wireHolder v1 (Autodesk Fusion 360 design; units mm, degrees)
Autodesk Fusion 360 part; units mm, degrees
sketch "Sketch1" plane through (0, 0, 0) normal (0, 0, 1) x (1, 0, 0)
  line L0 (0, 0) -> (40, 0)
  line L1 (40, 0) -> (40, 20)
  line L2 (40, 20) -> (0, 20)
  line L3 (0, 20) -> (0, 0)
  line L4 (5, 15) -> (35, 15)
  line L5 (35, 15) -> (35, 5)
  line L6 (35, 5) -> (5, 5)
  line L7 (5, 5) -> (5, 15)
  line L8 (16, 0) -> (16, 20)
  line L9 (24, 0) -> (24, 20)
  dimension "d1" = 40
  dimension "d2" = 20
  dimension "d3" = 5
  dimension "d4" = 5
  dimension "d5" = 10
  dimension "d6" = 5
  dimension "d16" = 16
  dimension "d17" = 8
  constraint horizontal L0
  constraint vertical L1
  constraint horizontal L2
  constraint vertical L3
  constraint coincident L0.start L3.end
  constraint horizontal L4
  constraint vertical L5
  constraint horizontal L6
  constraint vertical L7
  constraint coincident L0 L8.start
  constraint coincident L2 L8.end
  constraint perpendicular L2 L8
  constraint coincident L0 L9.start
  constraint coincident L2 L9.end
  constraint perpendicular L2 L9
  measures "d1" distance of L0.start L0.end
  measures "d2" distance of L0.start L2.end
  measures "d3" distance of L0 L6
  measures "d4" distance of L1 L5
  measures "d5" distance of L4 L6
  measures "d6" distance of L3 L7
  measures "d16" distance of L1 L9
  measures "d17" distance of L8 L9
extrude "Extrude1" add sketch "Sketch1" along normal blind 2
extrude "Extrude2" add sketch "Sketch1" along normal blind 20 contours L4 L6 L8 L9 | L4 L6 L7 L8 | L4 L5 L6 L9
fillet "Fillet1" radius 15 2 edges at (5, 10, 20) (35, 10, 20)
sketch "Sketch2" plane through (0, 5, 0) normal (0, -1, 0) x (1, 0, 0)
  arc A0 (35, 5) -> (5, 5) centre (20, 5) ccw
  line L0 (5, 5) -> (5, 2)
  line L1 (5, 2) -> (35, 2)
  line L2 (35, 2) -> (35, 5)
  line L3 (8, 5.1637) -> (32, 5.1637)
  arc A1 (32, 5.1637) -> (8, 5.1637) centre (20, 6.2496) ccw
  line L4 (8, 5.1637) -> (8, 2)
  line L5 (32, 5.1637) -> (32, 2)
  line L6 (8, 2) -> (32, 2)
  dimension "d13" = 3
  dimension "d14" = 3
  constraint parallel L1 L3
  constraint coincident L1 L4.end
  constraint perpendicular L1 L4
  constraint coincident L1 L5.end
  constraint perpendicular L1 L5
  measures "d13" distance of L0 L4
  measures "d14" distance of L2 L5
extrude "Extrude3" cut sketch "Sketch2" against normal through all contours L1 L3 L4 L5 L6 | L3 A1
extrude "Extrude4" cut sketch "Sketch1" along normal blind 2 contours L0 L6 L8 L9 | L4 L6 L8 L9 | L2 L4 L8 L9
